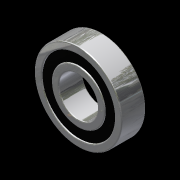
# Autodesk Inventor part: R8-2RS
Saved by Autodesk Inventor 2014 SP1 (Build 180222100, 222)
## iProperties
Created: 2014-04-23
Part Number: R8-2RS
Material: Generic
Document SubType Name: Modeling
Designer: Rauhul Varma
Density: 1 g/cm^3
Appearance: Default
Author: Rauhul Varma
Autodesk Inventor part; units mm, degrees
ref_plane "YZ Plane" through (0, 0, 0) normal (1, 0, 0) x (0, 1, 0)
ref_plane "XZ Plane" through (0, 0, 0) normal (0, 1, 0) x (-1, 0, 0)
ref_plane "XY Plane" through (0, 0, 0) normal (0, 0, 1) x (1, 0, 0)
sketch "Sketch1" plane through (0, 0, 0) normal (0, 0, 1) x (1, 0, 0)
  circle A0 centre (0, 0) radius 6.35
  circle A1 centre (0, 0) radius 14.2875
  circle A2 centre (0, 0) radius 8.7313
  circle A3 centre (0, 0) radius 11.9062
  dimension "d0" = 12.7
  dimension "d1" = 28.575
  dimension "d2" = 17.4625
  dimension "d3" = 2.3813
  constraints: 4 centre point, 4 coincident
  measures "d0" diameter of A0
  measures "d1" diameter of A1
  measures "d2" diameter of A2
  measures "d3" radial gap between concentric circles of A1 A3
extrude "Extrusion1" add sketch "Sketch1" along normal mid plane 7.9375
extrude "Extrusion2" add sketch "Sketch1" along normal mid plane 7.1437 contours A3
fillet "Fillet1" radius 0.3969 8 edges at (-6.35, 0, 3.9688) (-8.7313, 0, 3.9688) (-11.9062, 0, 3.9688) (-14.2875, 0, 3.9688) (-14.2875, 0, -3.9688) (-11.9062, 0, -3.9688) (-8.7313, 0, -3.9688) (-6.35, 0, -3.9688)
equation "\"d2\" = d0 + 2 * d3"
body "Solid1"
